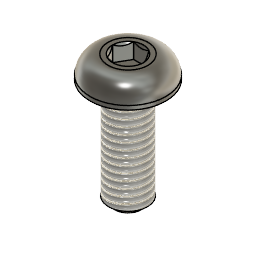
M3 Parametric BHCS (Autodesk Fusion 360 design; units mm, degrees)
part number: M3x8mm BHCS
Autodesk Fusion 360 part; units mm, degrees
sketch "Sketch1" plane through (0, 0, 0) normal (0, 1, 0) x (1, 0, 0)
  line L0 (0, 0) -> (1, 0)
  line L1 (1, 0) -> (1.5, -0.4641)
  line L2 (1.5, -0.4641) -> (1.5, -8)
  line L3 (1.5, -8) -> (2.85, -8)
  line L4 (2.85, -8) -> (2.85, -8.3)
  arc A0 (1.5, -9.65) -> (2.85, -8.3) centre (1.5, -8.3) ccw
  line L5 (1.5, -9.65) -> (0, -9.65)
  line L6 (0, -9.65) -> (0, 0)
  line L7 (1.1545, -9.65) -> (0, -8.4955)
  dimension "d2" = 8
  dimension "d3" = 0.5
  dimension "d4" = 1.5
  dimension "d5" = 1.5
  dimension "d6" = 2.85
  dimension "d7" = 1.65
  dimension "d11" = 1.1545
  dimension "d12" = 45
  constraint coincident L0.start L6.end
  constraint horizontal L0
  constraint perpendicular L0 L2
  constraint perpendicular L2 L3
  constraint perpendicular L3 L4
  constraint tangent L4 A0
  constraint perpendicular L4 L5
  constraint vertical L6
  constraint tangent A0 L5
  constraint coincident L5 L7.start
  constraint coincident L6 L7.end
  measures "d2" distance of L0 L3
  measures "d3" horizontal distance of L0.end L1.end
  measures "d4" distance of L2 L6
  measures "d5" distance of A0.start L5.end
  measures "d6" distance of L4 L6
  measures "d7" distance of L3 L5
  measures "d11" distance of L6 L7.start
  measures "d12" angle of L5 L7
revolve "Revolve1" add sketch "Sketch1" angle 360 about axis through (0, 0, 9.65) along (0, 0, -1) contours L0 L1 L2 L3 L4 A0 L5 L6 L7
sketch "Sketch2" plane through (0, 0, 9.65) normal (0, 0, 1) x (-1, 0, 0)
  circle A0 centre (0, 0) radius 1.5
  circle A1 centre (0, 0) radius 1.1545
  line L0 (-0.5774, 1) -> (-1.1547, 0)
  line L1 (-1.1547, 0) -> (-0.5774, -1)
  line L2 (-0.5774, -1) -> (0.5774, -1)
  line L3 (0.5774, -1) -> (1.1547, 0)
  line L4 (1.1547, 0) -> (0.5774, 1)
  line L5 (0.5774, 1) -> (-0.5774, 1)
  dimension "d14" = 1
  constraint coincident A0.centre A1.centre
  constraint horizontal L5
  measures "d14" distance of A0.centre L5
extrude "Extrude1" cut sketch "Sketch2" against normal blind 1.155 contours L0 L1 L2 L3 L4 L5
thread "Thread1" "ISO Metric profile 3.0 M3x0.5 6g" major diameter 2.927 minor diameter 2.3555 pitch 0.5 angle 60 resizes the face on face at (1.4981, 0.0748, 5.488)
equation "Length = 8 mm"
equation "d2 = Length"
equation "d4 = ( 3 / 2 ) * 1 mm"
equation "d5 = ( 3 / 2 ) * 1 mm"
equation "d6 = Head_Diameter / 2"
equation "d7 = Head_Length"
equation "d11 = 2.309 mm / 2"
equation "Head_Length = 1.65 mm"
equation "Head_Diameter = 5.7 mm"
